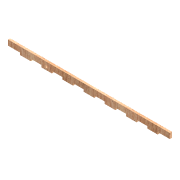
# Autodesk Inventor part: voorzijde onderkant elektrobox v2
Saved by Autodesk Inventor 2020.3 (Build 243373000, 373)
## iProperties
Created: 2020-11-26
Part Number: voorzijde onderkant elektrobox v2
Material: Wood (Birch)
Document SubType Name: Sheet Metal
Designer: Svend
Density: 0.55 g/cm^3
Sheet Metal Rule: Default_mm
Appearance: Birch - Natural Polished
Author: Svend
Autodesk Inventor part; units mm, degrees
ref_plane "YZ Plane" through (0, 0, 0) normal (1, 0, 0) x (0, 1, 0)
ref_plane "XZ Plane" through (0, 0, 0) normal (0, 1, 0) x (-1, 0, 0)
ref_plane "XY Plane" through (0, 0, 0) normal (0, 0, 1) x (1, 0, 0)
ref_plane "Work Plane1" through (0, 0, 0) normal (0, 0, 1) x (1, 0, 0)
sketch "Sketch1" plane through (0, 0, 0) normal (0, 0, 1) x (1, 0, 0)
  line L0 (-40, 0) -> (-40, 6)
  line L1 (-40, 6) -> (-34, 6)
  line L2 (0, 6) -> (-34, 6)
  line L3 (0, 6) -> (30, 6)
  line L4 (60, 6) -> (30, 6)
  line L5 (60, 6) -> (90, 6)
  line L6 (120, 6) -> (90, 6)
  line L7 (120, 6) -> (150, 6)
  line L8 (150, 6) -> (150, 0)
  line L9 (150, 0) -> (180, 0)
  line L10 (180, 0) -> (180, 6)
  line L11 (180, 6) -> (150, 6)
  line L12 (180, 6) -> (210, 6)
  line L13 (180, 0) -> (180, 6)
  line L14 (210, 0) -> (180, 0)
  line L15 (210, 0) -> (210, 6)
  line L16 (240, 0) -> (240, 6)
  line L17 (240, 6) -> (210, 6)
  line L18 (210, 6) -> (210, 0)
  line L19 (210, 0) -> (240, 0)
  line L20 (120, 6) -> (150, 6)
  line L21 (120, 0) -> (120, 6)
  line L22 (150, 0) -> (120, 0)
  line L23 (150, 0) -> (150, 6)
  line L24 (60, 6) -> (90, 6)
  line L25 (60, 0) -> (60, 6)
  line L26 (90, 0) -> (60, 0)
  line L27 (90, 0) -> (90, 6)
  line L28 (90, 6) -> (90, 0)
  line L29 (90, 0) -> (120, 0)
  line L30 (120, 0) -> (120, 6)
  line L31 (120, 6) -> (90, 6)
  line L32 (30, 6) -> (30, 0)
  line L33 (30, 0) -> (60, 0)
  line L34 (60, 0) -> (60, 6)
  line L35 (60, 6) -> (30, 6)
  line L36 (-34, 6) -> (-34, 0)
  line L37 (-34, 0) -> (0, 0)
  line L38 (0, 0) -> (0, 6)
  line L39 (0, 6) -> (-34, 6)
  line L40 (240, 0) -> (240, 6)
  line L41 (240, 6) -> (210, 6)
  line L42 (210, 6) -> (210, 0)
  line L43 (210, 0) -> (240, 0)
  line L44 (150, 6) -> (150, 0)
  line L45 (150, 0) -> (180, 0)
  line L46 (180, 0) -> (180, 6)
  line L47 (180, 6) -> (150, 6)
  line L48 (90, 6) -> (90, 0)
  line L49 (90, 0) -> (120, 0)
  line L50 (120, 0) -> (120, 6)
  line L51 (120, 6) -> (90, 6)
  line L52 (240, 6) -> (270, 6)
  line L53 (240, 0) -> (240, 6)
  line L54 (270, 0) -> (240, 0)
  line L55 (270, 0) -> (270, 6)
  line L56 (300, 0) -> (300, 6)
  line L57 (300, 6) -> (270, 6)
  line L58 (270, 6) -> (270, 0)
  line L59 (270, 0) -> (300, 0)
  line L60 (300, 6) -> (330, 6)
  line L61 (300, 0) -> (300, 6)
  line L62 (330, 0) -> (300, 0)
  line L63 (330, 0) -> (330, 6)
  line L64 (360, 0) -> (360, 6)
  line L65 (360, 6) -> (330, 6)
  line L66 (330, 6) -> (330, 0)
  line L67 (330, 0) -> (360, 0)
  line L68 (360, 6) -> (390, 6)
  line L69 (360, 0) -> (360, 6)
  line L70 (390, 0) -> (360, 0)
  line L71 (390, 0) -> (390, 6)
  line L72 (424, 0) -> (424, 6)
  line L73 (424, 6) -> (390, 6)
  line L74 (390, 6) -> (390, 0)
  line L75 (390, 0) -> (424, 0)
  line L76 (424, 6) -> (430, 6)
  line L77 (424, 0) -> (424, 6)
  line L78 (430, 0) -> (424, 0)
  line L79 (430, 6) -> (430, 0)
  line L80 (-40, 6) -> (-40, 21)
  line L81 (-40, 21) -> (430, 21)
  line L82 (430, 21) -> (430, 6)
  line L83 (0, 6) -> (30, 6)
  line L84 (0, 0) -> (0, 6)
  line L85 (30, 0) -> (0, 0)
  line L86 (30, 0) -> (30, 6)
  line L87 (-40, 6) -> (-34, 6)
  line L88 (-40, 0) -> (-40, 6)
  line L89 (-34, 0) -> (-40, 0)
  line L90 (-34, 0) -> (-34, 6)
  line L91 (-34, 6) -> (-34, 21)
  line L92 (424, 6) -> (424, 21)
  dimension "d0" = 15
  measures "d0" distance of L0.end L80.end
extrude "Plate1" add sketch "Sketch1" along normal blind 6 contours L91 L81 L92 L73 L68 L65 L60 L57 L52 L17 L12 L11 L7 L6 L5 L4 L3 L2 | L38 L3 L32 L85 | L25 L5 L27 L26 | L71 L70 L64 L68 | L21 L7 L8 L22 | L63 L62 L56 L60 | L10 L12 L15 L14 | L55 L54 L16 L52
sketch "Sketch2" plane through (0, 0, 6) normal (0, 0, 1) x (1, 0, 0)
  line L0 (71.2707, 6) -> (65.2707, 6) projected
  line L1 (83.7293, 6) -> (77.7293, 6) projected
  line L2 (-34, 6) -> (-34, 21) projected
  line L3 (0, 6) -> (-34, 6) projected
  line L4 (0, 0) -> (0, 6) projected
  line L5 (30, 0) -> (0, 0) projected
  line L6 (30, 6) -> (30, 0) projected
  line L7 (60, 6) -> (30, 6) projected
  line L8 (60, 0) -> (60, 6) projected
  line L9 (90, 0) -> (60, 0) projected
  line L10 (90, 6) -> (90, 0) projected
  line L11 (120, 6) -> (90, 6) projected
  line L12 (120, 0) -> (120, 6) projected
  line L13 (150, 0) -> (120, 0) projected
  line L14 (150, 6) -> (150, 0) projected
  line L15 (180, 6) -> (150, 6) projected
  line L16 (180, 0) -> (180, 6) projected
  line L17 (210, 0) -> (180, 0) projected
  line L18 (210, 6) -> (210, 0) projected
  line L19 (240, 6) -> (210, 6) projected
  line L20 (240, 0) -> (240, 6) projected
  line L21 (270, 0) -> (240, 0) projected
  line L22 (270, 6) -> (270, 0) projected
  line L23 (300, 6) -> (270, 6) projected
  line L24 (300, 0) -> (300, 6) projected
  line L25 (330, 0) -> (300, 0) projected
  line L26 (330, 6) -> (330, 0) projected
  line L27 (360, 6) -> (330, 6) projected
  line L28 (360, 0) -> (360, 6) projected
  line L29 (390, 0) -> (360, 0) projected
  line L30 (390, 6) -> (390, 0) projected
  line L31 (424, 6) -> (390, 6) projected
  line L32 (424, 21) -> (424, 6) projected
  line L33 (-34, 21) -> (424, 21) projected
  line L34 (77.6, 6) -> (71.4, 6)
  line L35 (71.4, 6) -> (71.4, 12.2)
  line L36 (71.4, 12.2) -> (77.6, 12.2)
  line L37 (77.6, 12.2) -> (77.6, 6)
  line L38 (71.2707, 6) -> (77.7293, 6) construction
  point P0 (0, 0)
  point P1 (74.5, 6)
  point P2 (74.5, 6)
  dimension "d2" = 6.2
  dimension "d3" = 6.2
  constraints: 10 end point, 2 collinear, 2 midpoint, 2 parallel, 1 coincident, 1 horizontal, 1 perpendicular
  measures "d2" distance of L35.end L36.end
  measures "d3" distance of L36.end L34.start
extrude "Cut1" cut sketch "Sketch2" against normal blind 6 contours L34 L35 L36 L37
equation "\"d3\" = d2"
equation "\"d4\" = Thickness"
equation "\"d1\" = Thickness"
equation "\"BendRadius\" = Thickness"
equation "\"BendReliefWidth\" = Thickness"
equation "\"BendReliefDepth\" = 0.5 * Thickness"
equation "\"CornerReliefSize\" = 4 * Thickness"
equation "\"MinimumRemnant\" = 2 * Thickness"
equation "\"TransitionRadius\" = BendRadius"
equation "\"JacobiRadiusSize\" = BendRadius"
equation "\"GapSize\" = Thickness"
equation "\"Thickness\" = 6"
body "Solid1"
